Autodesk Fusion 360 part; units mm, degrees
note: some values were not read from the file. Set by a fixed rule: which sketch regions a step uses.
(part 2 of 2)
sketch "bottom inner" plane through (0, 3.175, 0) normal (0, 1, 0) x (-1, 0, 0)
  line L0 (-22.86, -3.175) -> (-24.3417, -3.175)
  line L1 (-24.3417, -3.175) -> (-24.3417, -4.8013)
  arc A0 (-32.8083, -4.8013) -> (-24.3417, -4.8013) centre (-28.575, -4.8013) ccw
  line L2 (-32.8083, -4.8013) -> (-32.8083, -3.175)
  line L3 (-32.8083, -3.175) -> (-53.975, -3.175)
  line L4 (-53.975, -3.175) -> (-53.975, -88.9)
  line L5 (-53.975, -88.9) -> (-32.8083, -88.9)
  line L6 (-32.8083, -88.9) -> (-32.8083, -87.2737)
  arc A1 (-24.3417, -87.2737) -> (-32.8083, -87.2737) centre (-28.575, -87.2737) ccw
  line L7 (-24.3417, -87.2737) -> (-24.3417, -88.9)
  line L8 (-24.3417, -88.9) -> (-3.175, -88.9)
  line L9 (-3.175, -88.9) -> (-3.175, -3.175)
  line L10 (-3.175, -3.175) -> (-7.62, -3.175)
  line L11 (-7.62, -3.175) -> (-7.62, 0)
  line L12 (-7.62, 0) -> (-22.86, 0)
  line L13 (-22.86, 0) -> (-22.86, -3.175)
  spline S0 degree 3 poles (-12.8176, -66.9854) (-12.904, -65.2247) (-13.5003, -63.4767) (-14.5669, -61.8591) knots 0 0 0 0 1 1 1 1
  spline S1 degree 3 poles (-14.5669, -61.8591) (-15.5301, -60.4001) (-16.8758, -59.1069) (-18.9651, -57.638) knots 0 0 0 0 1 1 1 1
  spline S2 degree 3 poles (-18.9651, -57.638) (-20.4751, -56.5756) (-21.3505, -55.9099) (-21.7145, -55.5472) knots 0 0 0 0 1 1 1 1
  spline S3 degree 3 poles (-21.7145, -55.5472) (-22.6537, -54.6081) (-23.284, -53.0854) (-23.7954, -50.5229) knots 0 0 0 0 1 1 1 1
  spline S4 degree 3 poles (-23.7954, -50.5229) (-23.8903, -50.0428) (-23.9837, -49.5059) (-24.1141, -48.6787) knots 0 0 0 0 1 1 1 1
  spline S5 degree 3 poles (-24.1141, -48.6787) (-24.3634, -47.1007) (-24.4795, -46.6673) (-24.6552, -46.6673) knots 0 0 0 0 1 1 1 1
  spline S6 degree 3 poles (-24.6552, -46.6673) (-24.8181, -46.6673) (-24.8521, -46.8953) (-24.8393, -47.8854) knots 0 0 0 0 1 1 1 1
  spline S7 degree 3 poles (-24.8393, -47.8854) (-24.8308, -48.5059) (-24.8209, -48.7254) (-24.7727, -49.4082) knots 0 0 0 0 1 1 1 1
  spline S8 degree 3 poles (-24.7727, -49.4082) (-24.6821, -50.6674) (-24.5574, -51.5626) (-24.3393, -52.5174) knots 0 0 0 0 1 1 1 1
  spline S9 degree 3 poles (-24.3393, -52.5174) (-23.9894, -54.0358) (-23.4724, -55.2314) (-22.8817, -55.8844) knots 0 0 0 0 1 1 1 1
  spline S10 degree 3 poles (-22.8817, -55.8844) (-22.5644, -56.2356) (-21.6097, -56.9666) (-20.4524, -57.7485) knots 0 0 0 0 1 1 1 1
  spline S11 degree 3 poles (-20.4524, -57.7485) (-19.8221, -58.1748) (-19.4708, -58.4227) (-19.0997, -58.7003) knots 0 0 0 0 1 1 1 1
  spline S12 degree 3 poles (-19.0997, -58.7003) (-17.6733, -59.7726) (-16.6548, -60.7967) (-15.8913, -61.9299) knots 0 0 0 0 1 1 1 1
  spline S13 degree 3 poles (-15.8913, -61.9299) (-15.006, -63.2459) (-14.4352, -64.6043) (-14.2128, -65.9244) knots 0 0 0 0 1 1 1 1
  spline S14 degree 3 poles (-14.2128, -65.9244) (-14.0372, -66.9741) (-14.0896, -67.9543) (-14.3714, -68.8282) knots 0 0 0 0 1 1 1 1
  spline S15 degree 3 poles (-14.3714, -68.8282) (-14.591, -69.5082) (-14.9352, -70.079) (-15.4154, -70.5564) knots 0 0 0 0 1 1 1 1
  spline S16 degree 3 poles (-15.4154, -70.5564) (-15.6321, -70.7731) (-15.7752, -70.8892) (-16.0188, -71.0521) knots 0 0 0 0 1 1 1 1
  spline S17 degree 3 poles (-16.0188, -71.0521) (-16.6279, -71.4572) (-17.3007, -71.6924) (-18.1365, -71.7901) knots 0 0 0 0 1 1 1 1
  spline S18 degree 3 poles (-18.1365, -71.7901) (-18.441, -71.827) (-19.162, -71.827) (-19.4396, -71.7915) knots 0 0 0 0 1 1 1 1
  spline S19 degree 3 poles (-19.4396, -71.7915) (-21.0176, -71.5876) (-22.8449, -70.6923) (-24.4087, -69.3552) knots 0 0 0 0 1 1 1 1
  spline S20 degree 3 poles (-24.4087, -69.3552) (-24.6452, -69.154) (-25.1283, -68.6823) (-25.3252, -68.46) knots 0 0 0 0 1 1 1 1
  spline S21 degree 3 poles (-25.3252, -68.46) (-25.8025, -67.9217) (-26.1722, -67.3636) (-26.379, -66.8692) knots 0 0 0 0 1 1 1 1
  line L14 (-26.379, -66.8692) -> (-26.4173, -66.78)
  line L15 (-26.4173, -66.78) -> (-26.304, -66.5505)
  spline S22 degree 3 poles (-26.304, -66.5505) (-26.1793, -66.2984) (-26.1141, -66.1312) (-26.0391, -65.8706) knots 0 0 0 0 1 1 1 1
  spline S23 degree 3 poles (-26.0391, -65.8706) (-25.8096, -65.0717) (-25.7558, -63.964) (-25.9144, -63.2558) knots 0 0 0 0 1 1 1 1
  spline S24 degree 3 poles (-25.9144, -63.2558) (-25.9654, -63.0277) (-26.0334, -62.8422) (-26.1595, -62.5815) knots 0 0 0 0 1 1 1 1
  spline S25 degree 3 poles (-26.1595, -62.5815) (-26.4116, -62.0631) (-26.7771, -61.5319) (-27.0165, -61.3407) knots 0 0 0 0 1 1 1 1
  spline S26 degree 3 poles (-27.0165, -61.3407) (-27.1227, -61.2543) (-27.2332, -61.2217) (-27.389, -61.2316) knots 0 0 0 0 1 1 1 1
  spline S27 degree 3 poles (-27.389, -61.2316) (-27.593, -61.2444) (-27.7502, -61.3648) (-27.8777, -61.6056) knots 0 0 0 0 1 1 1 1
  spline S28 degree 3 poles (-27.8777, -61.6056) (-28.042, -61.9186) (-28.1227, -62.3166) (-28.1397, -62.9002) knots 0 0 0 0 1 1 1 1
  spline S29 degree 3 poles (-28.1397, -62.9002) (-28.1553, -63.447) (-28.0873, -64.0915) (-27.9513, -64.7063) knots 0 0 0 0 1 1 1 1
  spline S30 degree 3 poles (-27.9513, -64.7063) (-27.855, -65.1411) (-27.5915, -66.1808) (-27.5207, -66.4103) knots 0 0 0 0 1 1 1 1
  spline S31 degree 3 poles (-27.5207, -66.4103) (-27.4357, -66.6851) (-27.4244, -66.644) (-27.6397, -66.8593) knots 0 0 0 0 1 1 1 1
  spline S32 degree 3 poles (-27.6397, -66.8593) (-28.0774, -67.2956) (-28.7757, -67.6809) (-29.8763, -68.0903) knots 0 0 0 0 1 1 1 1
  spline S33 degree 3 poles (-29.8763, -68.0903) (-30.4599, -68.307) (-30.6455, -68.3594) (-31.0336, -68.416) knots 0 0 0 0 1 1 1 1
  spline S34 degree 3 poles (-31.0336, -68.416) (-32.0832, -68.569) (-33.8694, -68.5223) (-35.1556, -68.3098) knots 0 0 0 0 1 1 1 1
  spline S35 degree 3 poles (-35.1556, -68.3098) (-35.6202, -68.2333) (-35.8681, -68.171) (-36.2817, -68.0251) knots 0 0 0 0 1 1 1 1
  spline S36 degree 3 poles (-36.2817, -68.0251) (-38.1416, -67.3707) (-39.8314, -66.2177) (-40.5808, -65.0915) knots 0 0 0 0 1 1 1 1
  spline S37 degree 3 poles (-40.5808, -65.0915) (-41.0114, -64.4442) (-41.3839, -63.2175) (-41.5326, -61.9512) knots 0 0 0 0 1 1 1 1
  spline S38 degree 3 poles (-41.5326, -61.9512) (-41.561, -61.7061) (-41.5652, -61.6084) (-41.5652, -61.0871) knots 0 0 0 0 1 1 1 1
  spline S39 degree 3 poles (-41.5652, -61.0871) (-41.5652, -60.4894) (-41.5581, -60.369) (-41.5001, -59.8973) knots 0 0 0 0 1 1 1 1
  spline S40 degree 3 poles (-41.5001, -59.8973) (-41.2522, -57.8944) (-40.3626, -56.3405) (-38.9872, -55.5047) knots 0 0 0 0 1 1 1 1
  spline S41 degree 3 poles (-38.9872, -55.5047) (-38.7846, -55.3815) (-38.279, -55.1336) (-38.0835, -55.0614) knots 0 0 0 0 1 1 1 1
  spline S42 degree 3 poles (-38.0835, -55.0614) (-37.7676, -54.9438) (-37.5509, -54.9041) (-37.0778, -54.8801) knots 0 0 0 0 1 1 1 1
  spline S43 degree 3 poles (-37.0778, -54.8801) (-36.5537, -54.8532) (-36.2166, -54.8857) (-35.293, -55.0515) knots 0 0 0 0 1 1 1 1
  spline S44 degree 3 poles (-35.293, -55.0515) (-34.4573, -55.203) (-34.1343, -55.2342) (-33.8439, -55.1931) knots 0 0 0 0 1 1 1 1
  spline S45 degree 3 poles (-33.8439, -55.1931) (-33.6145, -55.162) (-33.4955, -55.0925) (-33.2561, -54.8546) knots 0 0 0 0 1 1 1 1
  spline S46 degree 3 poles (-33.2561, -54.8546) (-33.0535, -54.6534) (-33.0025, -54.5642) (-33.0025, -54.414) knots 0 0 0 0 1 1 1 1
  spline S47 degree 3 poles (-33.0025, -54.414) (-33.0025, -54.1817) (-33.1952, -53.7851) (-33.5054, -53.3814) knots 0 0 0 0 1 1 1 1
  spline S48 degree 3 poles (-33.5054, -53.3814) (-33.5564, -53.3148) (-33.5975, -53.2568) (-33.5975, -53.2511) knots 0 0 0 0 1 1 1 1
  spline S49 degree 3 poles (-33.5975, -53.2511) (-33.5975, -53.227) (-33.4785, -53.1817) (-33.3609, -53.1619) knots 0 0 0 0 1 1 1 1
  spline S50 degree 3 poles (-33.3609, -53.1619) (-33.2901, -53.1491) (-33.0719, -53.135) (-32.8538, -53.1265) knots 0 0 0 0 1 1 1 1
  spline S51 degree 3 poles (-32.8538, -53.1265) (-32.3552, -53.1095) (-32.1583, -53.074) (-31.9218, -52.9551) knots 0 0 0 0 1 1 1 1
  spline S52 degree 3 poles (-31.9218, -52.9551) (-31.6144, -52.8007) (-31.3622, -52.5018) (-31.2121, -52.1137) knots 0 0 0 0 1 1 1 1
  spline S53 degree 3 poles (-31.2121, -52.1137) (-31.1384, -51.921) (-31.1144, -51.7893) (-31.1144, -51.5683) knots 0 0 0 0 1 1 1 1
  spline S54 degree 3 poles (-31.1144, -51.5683) (-31.1158, -51.3417) (-31.1455, -51.1759) (-31.2319, -50.9238) knots 0 0 0 0 1 1 1 1
  spline S55 degree 3 poles (-31.2319, -50.9238) (-31.3183, -50.6773) (-31.3835, -50.5569) (-31.5407, -50.3657) knots 0 0 0 0 1 1 1 1
  spline S56 degree 3 poles (-31.5407, -50.3657) (-31.5818, -50.3161) (-31.6101, -50.2708) (-31.6045, -50.2651) knots 0 0 0 0 1 1 1 1
  spline S57 degree 3 poles (-31.6045, -50.2651) (-31.5988, -50.2595) (-31.5336, -50.2156) (-31.4614, -50.166) knots 0 0 0 0 1 1 1 1
  spline S58 degree 3 poles (-31.4614, -50.166) (-30.9741, -49.8359) (-31.0166, -49.3473) (-31.5804, -48.8062) knots 0 0 0 0 1 1 1 1
  spline S59 degree 3 poles (-31.5804, -48.8062) (-31.807, -48.588) (-32.0563, -48.401) (-32.4855, -48.1248) knots 0 0 0 0 1 1 1 1
  spline S60 degree 3 poles (-32.4855, -48.1248) (-32.7929, -47.9294) (-32.9147, -47.8344) (-33.0734, -47.673) knots 0 0 0 0 1 1 1 1
  spline S61 degree 3 poles (-33.0734, -47.673) (-33.2164, -47.5285) (-33.283, -47.4307) (-33.3283, -47.3004) knots 0 0 0 0 1 1 1 1
  spline S62 degree 3 poles (-33.3283, -47.3004) (-33.4062, -47.078) (-33.3085, -46.8812) (-33.0578, -46.7622) knots 0 0 0 0 1 1 1 1
  spline S63 degree 3 poles (-33.0578, -46.7622) (-32.8283, -46.6517) (-32.6583, -46.6262) (-32.096, -46.6106) knots 0 0 0 0 1 1 1 1
  spline S64 degree 3 poles (-32.096, -46.6106) (-31.841, -46.6035) (-31.6243, -46.5908) (-31.5903, -46.5823) knots 0 0 0 0 1 1 1 1
  spline S65 degree 3 poles (-31.5903, -46.5823) (-31.4727, -46.5483) (-31.4302, -46.4562) (-31.4302, -46.2366) knots 0 0 0 0 1 1 1 1
  spline S66 degree 3 poles (-31.4302, -46.2366) (-31.4302, -46.0058) (-31.477, -45.8726) (-31.596, -45.7593) knots 0 0 0 0 1 1 1 1
  spline S67 degree 3 poles (-31.596, -45.7593) (-31.688, -45.6715) (-31.7872, -45.6049) (-32.0818, -45.4406) knots 0 0 0 0 1 1 1 1
  spline S68 degree 3 poles (-32.0818, -45.4406) (-32.341, -45.2961) (-32.6371, -45.1091) (-32.783, -44.9986) knots 0 0 0 0 1 1 1 1
  spline S69 degree 3 poles (-32.783, -44.9986) (-32.9218, -44.8924) (-33.1513, -44.6601) (-33.2263, -44.551) knots 0 0 0 0 1 1 1 1
  spline S70 degree 3 poles (-33.2263, -44.551) (-33.3793, -44.3301) (-33.4204, -44.204) (-33.4204, -43.9618) knots 0 0 0 0 1 1 1 1
  spline S71 degree 3 poles (-33.4204, -43.9618) (-33.419, -43.8329) (-33.4119, -43.762) (-33.3935, -43.6997) knots 0 0 0 0 1 1 1 1
  spline S72 degree 3 poles (-33.3935, -43.6997) (-33.2915, -43.3583) (-33.0394, -43.1898) (-32.4784, -43.0835) knots 0 0 0 0 1 1 1 1
  spline S73 degree 3 poles (-32.4784, -43.0835) (-32.147, -43.0212) (-31.9317, -42.9362) (-31.7929, -42.8116) knots 0 0 0 0 1 1 1 1
  spline S74 degree 3 poles (-31.7929, -42.8116) (-31.5832, -42.6246) (-31.5903, -42.364) (-31.8113, -42.16) knots 0 0 0 0 1 1 1 1
  spline S75 degree 3 poles (-31.8113, -42.16) (-31.977, -42.0056) (-32.2532, -41.8243) (-32.7122, -41.5679) knots 0 0 0 0 1 1 1 1
  spline S76 degree 3 poles (-32.7122, -41.5679) (-33.0875, -41.3583) (-33.2717, -41.2393) (-33.3921, -41.1274) knots 0 0 0 0 1 1 1 1
  spline S77 degree 3 poles (-33.3921, -41.1274) (-33.5408, -40.9871) (-33.5451, -40.9135) (-33.4077, -40.8512) knots 0 0 0 0 1 1 1 1
  spline S78 degree 3 poles (-33.4077, -40.8512) (-33.2858, -40.7959) (-33.0946, -40.7747) (-32.5634, -40.7605) knots 0 0 0 0 1 1 1 1
  spline S79 degree 3 poles (-32.5634, -40.7605) (-32.2943, -40.7534) (-32.0209, -40.7407) (-31.9543, -40.7322) knots 0 0 0 0 1 1 1 1
  spline S80 degree 3 poles (-31.9543, -40.7322) (-31.4926, -40.6727) (-31.2815, -40.565) (-31.2631, -40.3795) knots 0 0 0 0 1 1 1 1
  spline S81 degree 3 poles (-31.2631, -40.3795) (-31.2447, -40.1882) (-31.4203, -39.9531) (-31.841, -39.599) knots 0 0 0 0 1 1 1 1
  spline S82 degree 3 poles (-31.841, -39.599) (-32.5082, -39.038) (-33.2462, -38.1329) (-33.5776, -37.4672) knots 0 0 0 0 1 1 1 1
  spline S83 degree 3 poles (-33.5776, -37.4672) (-33.7122, -37.1938) (-33.7448, -37.0748) (-33.7363, -36.8666) knots 0 0 0 0 1 1 1 1
  spline S84 degree 3 poles (-33.7363, -36.8666) (-33.732, -36.7575) (-33.7207, -36.6952) (-33.698, -36.6371) knots 0 0 0 0 1 1 1 1
  spline S85 degree 3 poles (-33.698, -36.6371) (-33.6074, -36.4034) (-33.3496, -36.2787) (-33.1059, -36.3524) knots 0 0 0 0 1 1 1 1
  spline S86 degree 3 poles (-33.1059, -36.3524) (-32.8113, -36.443) (-32.4317, -36.8354) (-32.2051, -37.283) knots 0 0 0 0 1 1 1 1
  spline S87 degree 3 poles (-32.2051, -37.283) (-32.1243, -37.4431) (-32.096, -37.5153) (-32.0096, -37.7788) knots 0 0 0 0 1 1 1 1
  spline S88 degree 3 poles (-32.0096, -37.7788) (-31.8778, -38.1811) (-31.7419, -38.4545) (-31.613, -38.5706) knots 0 0 0 0 1 1 1 1
  spline S89 degree 3 poles (-31.613, -38.5706) (-31.4996, -38.6726) (-31.3792, -38.725) (-31.2404, -38.7321) knots 0 0 0 0 1 1 1 1
  spline S90 degree 3 poles (-31.2404, -38.7321) (-31.0534, -38.742) (-30.9628, -38.6797) (-30.9628, -38.5409) knots 0 0 0 0 1 1 1 1
  spline S91 degree 3 poles (-30.9628, -38.5409) (-30.9628, -38.2406) (-31.6002, -36.6102) (-31.9274, -36.0762) knots 0 0 0 0 1 1 1 1
  spline S92 degree 3 poles (-31.9274, -36.0762) (-32.1399, -35.7277) (-32.4544, -35.4331) (-32.7801, -35.273) knots 0 0 0 0 1 1 1 1
  spline S93 degree 3 poles (-32.7801, -35.273) (-33.3212, -35.0081) (-33.8935, -35.0775) (-34.3015, -35.4543) knots 0 0 0 0 1 1 1 1
  spline S94 degree 3 poles (-34.3015, -35.4543) (-34.6442, -35.773) (-34.7774, -36.1895) (-34.7321, -36.8085) knots 0 0 0 0 1 1 1 1
  spline S95 degree 3 poles (-34.7321, -36.8085) (-34.6967, -37.3) (-34.5947, -37.6612) (-34.368, -38.0975) knots 0 0 0 0 1 1 1 1
  spline S96 degree 3 poles (-34.368, -38.0975) (-34.1825, -38.4545) (-33.9573, -38.7647) (-33.4771, -39.3298) knots 0 0 0 0 1 1 1 1
  spline S97 degree 3 poles (-33.4771, -39.3298) (-33.1173, -39.7534) (-33.0535, -39.8341) (-33.0649, -39.8511) knots 0 0 0 0 1 1 1 1
  spline S98 degree 3 poles (-33.0649, -39.8511) (-33.0691, -39.8582) (-33.1286, -39.8695) (-33.1966, -39.8738) knots 0 0 0 0 1 1 1 1
  spline S99 degree 3 poles (-33.1966, -39.8738) (-33.6895, -39.9134) (-33.9898, -40.0197) (-34.208, -40.2364) knots 0 0 0 0 1 1 1 1
  spline S100 degree 3 poles (-34.208, -40.2364) (-34.3794, -40.405) (-34.453, -40.5792) (-34.4516, -40.8172) knots 0 0 0 0 1 1 1 1
  spline S101 degree 3 poles (-34.4516, -40.8172) (-34.4516, -41.0381) (-34.3794, -41.2492) (-34.2292, -41.4744) knots 0 0 0 0 1 1 1 1
  spline S102 degree 3 poles (-34.2292, -41.4744) (-34.123, -41.6316) (-34.0068, -41.7563) (-33.7235, -42.0084) knots 0 0 0 0 1 1 1 1
  line L16 (-33.7235, -42.0084) -> (-33.4813, -42.2251)
  line L17 (-33.4813, -42.2251) -> (-33.7136, -42.4518)
  spline S103 degree 3 poles (-33.7136, -42.4518) (-33.9573, -42.6912) (-34.0578, -42.8172) (-34.1527, -43.0056) knots 0 0 0 0 1 1 1 1
  spline S104 degree 3 poles (-34.1527, -43.0056) (-34.293, -43.2804) (-34.3411, -43.5212) (-34.3298, -43.8683) knots 0 0 0 0 1 1 1 1
  spline S105 degree 3 poles (-34.3298, -43.8683) (-34.3185, -44.1785) (-34.266, -44.3995) (-34.1286, -44.6913) knots 0 0 0 0 1 1 1 1
  spline S106 degree 3 poles (-34.1286, -44.6913) (-34.0111, -44.9434) (-33.8793, -45.1332) (-33.5861, -45.4703) knots 0 0 0 0 1 1 1 1
  spline S107 degree 3 poles (-33.5861, -45.4703) (-33.3949, -45.6899) (-33.3637, -45.7352) (-33.3836, -45.772) knots 0 0 0 0 1 1 1 1
  spline S108 degree 3 poles (-33.3836, -45.772) (-33.3907, -45.7862) (-33.4941, -45.8868) (-33.6116, -45.993) knots 0 0 0 0 1 1 1 1
  spline S109 degree 3 poles (-33.6116, -45.993) (-33.9997, -46.3471) (-34.174, -46.5922) (-34.266, -46.9166) knots 0 0 0 0 1 1 1 1
  spline S110 degree 3 poles (-34.266, -46.9166) (-34.3057, -47.061) (-34.3085, -47.3203) (-34.2717, -47.4605) knots 0 0 0 0 1 1 1 1
  spline S111 degree 3 poles (-34.2717, -47.4605) (-34.2363, -47.5951) (-34.1343, -47.7962) (-34.0366, -47.9251) knots 0 0 0 0 1 1 1 1
  spline S112 degree 3 poles (-34.0366, -47.9251) (-33.8793, -48.1333) (-33.5946, -48.3741) (-33.2957, -48.5498) knots 0 0 0 0 1 1 1 1
  spline S113 degree 3 poles (-33.2957, -48.5498) (-33.2278, -48.5894) (-33.1173, -48.6546) (-33.0479, -48.6943) knots 0 0 0 0 1 1 1 1
  spline S114 degree 3 poles (-33.0479, -48.6943) (-32.7306, -48.8812) (-32.4048, -49.1631) (-32.3184, -49.3274) knots 0 0 0 0 1 1 1 1
  line L18 (-32.3184, -49.3274) -> (-32.2787, -49.4011)
  line L19 (-32.2787, -49.4011) -> (-32.3325, -49.4266)
  spline S115 degree 3 poles (-32.3325, -49.4266) (-32.3821, -49.4492) (-32.4629, -49.4507) (-33.2858, -49.4507) knots 0 0 0 0 1 1 1 1
  spline S116 degree 3 poles (-33.2858, -49.4507) (-34.1598, -49.4507) (-34.1867, -49.4521) (-34.2335, -49.479) knots 0 0 0 0 1 1 1 1
  spline S117 degree 3 poles (-34.2335, -49.479) (-34.327, -49.5342) (-34.361, -49.615) (-34.3624, -49.7835) knots 0 0 0 0 1 1 1 1
  spline S118 degree 3 poles (-34.3624, -49.7835) (-34.3638, -50.0555) (-34.2051, -50.1532) (-33.5451, -50.2864) knots 0 0 0 0 1 1 1 1
  spline S119 degree 3 poles (-33.5451, -50.2864) (-33.0974, -50.377) (-32.9218, -50.4309) (-32.6852, -50.5527) knots 0 0 0 0 1 1 1 1
  spline S120 degree 3 poles (-32.6852, -50.5527) (-32.3538, -50.7227) (-32.1427, -50.9493) (-32.0747, -51.2099) knots 0 0 0 0 1 1 1 1
  spline S121 degree 3 poles (-32.0747, -51.2099) (-32.0025, -51.4847) (-32.1243, -51.7709) (-32.3835, -51.9338) knots 0 0 0 0 1 1 1 1
  spline S122 degree 3 poles (-32.3835, -51.9338) (-32.5408, -52.0329) (-32.7107, -52.0882) (-32.9742, -52.1278) knots 0 0 0 0 1 1 1 1
  spline S123 degree 3 poles (-32.9742, -52.1278) (-33.606, -52.2227) (-33.9459, -52.3516) (-34.1655, -52.5825) knots 0 0 0 0 1 1 1 1
  spline S124 degree 3 poles (-34.1655, -52.5825) (-34.31, -52.7355) (-34.4034, -52.948) (-34.4148, -53.1562) knots 0 0 0 0 1 1 1 1
  spline S125 degree 3 poles (-34.4148, -53.1562) (-34.4247, -53.3078) (-34.4049, -53.3814) (-34.2845, -53.6364) knots 0 0 0 0 1 1 1 1
  spline S126 degree 3 poles (-34.2845, -53.6364) (-34.2363, -53.7412) (-34.1811, -53.8715) (-34.1655, -53.9268) knots 0 0 0 0 1 1 1 1
  spline S127 degree 3 poles (-34.1655, -53.9268) (-34.1371, -54.0188) (-34.1216, -54.1647) (-34.1386, -54.1817) knots 0 0 0 0 1 1 1 1
  spline S128 degree 3 poles (-34.1386, -54.1817) (-34.1513, -54.1945) (-34.5635, -54.084) (-34.7958, -54.0075) knots 0 0 0 0 1 1 1 1
  spline S129 degree 3 poles (-34.7958, -54.0075) (-35.0621, -53.9183) (-35.2803, -53.8616) (-35.5805, -53.8078) knots 0 0 0 0 1 1 1 1
  spline S130 degree 3 poles (-35.5805, -53.8078) (-36.361, -53.6647) (-36.8951, -53.6435) (-37.5353, -53.7299) knots 0 0 0 0 1 1 1 1
  spline S131 degree 3 poles (-37.5353, -53.7299) (-37.9192, -53.7809) (-38.3767, -53.8956) (-38.7535, -54.0344) knots 0 0 0 0 1 1 1 1
  spline S132 degree 3 poles (-38.7535, -54.0344) (-39.0269, -54.135) (-39.449, -54.3489) (-39.6742, -54.4976) knots 0 0 0 0 1 1 1 1
  spline S133 degree 3 poles (-39.6742, -54.4976) (-40.1218, -54.7951) (-40.5978, -55.2625) (-40.9958, -55.7965) knots 0 0 0 0 1 1 1 1
  spline S134 degree 3 poles (-40.9958, -55.7965) (-41.5992, -56.6054) (-42.0709, -57.5785) (-42.357, -58.6111) knots 0 0 0 0 1 1 1 1
  spline S135 degree 3 poles (-42.357, -58.6111) (-42.561, -59.3434) (-42.6531, -60.1707) (-42.6531, -61.2642) knots 0 0 0 0 1 1 1 1
  spline S136 degree 3 poles (-42.6531, -61.2642) (-42.6531, -62.1849) (-42.5879, -62.8209) (-42.4364, -63.3719) knots 0 0 0 0 1 1 1 1
  spline S137 degree 3 poles (-42.4364, -63.3719) (-42.2026, -64.2232) (-41.7437, -65.1624) (-41.1672, -65.9669) knots 0 0 0 0 1 1 1 1
  spline S138 degree 3 poles (-41.1672, -65.9669) (-40.5014, -66.899) (-39.7139, -67.6526) (-38.8852, -68.1497) knots 0 0 0 0 1 1 1 1
  spline S139 degree 3 poles (-38.8852, -68.1497) (-37.3101, -69.0945) (-34.0791, -69.8821) (-32.1668, -69.7858) knots 0 0 0 0 1 1 1 1
  spline S140 degree 3 poles (-32.1668, -69.7858) (-30.984, -69.7263) (-29.9047, -69.4444) (-28.8664, -68.9246) knots 0 0 0 0 1 1 1 1
  spline S141 degree 3 poles (-28.8664, -68.9246) (-28.3919, -68.688) (-28.0448, -68.4685) (-27.6624, -68.1625) knots 0 0 0 0 1 1 1 1
  spline S142 degree 3 poles (-27.6624, -68.1625) (-27.5646, -68.0846) (-27.4244, -67.9741) (-27.3507, -67.916) knots 0 0 0 0 1 1 1 1
  spline S143 degree 3 poles (-27.3507, -67.916) (-27.2771, -67.8579) (-27.1708, -67.7701) (-27.1156, -67.7205) knots 0 0 0 0 1 1 1 1
  spline S144 degree 3 poles (-27.1156, -67.7205) (-27.0589, -67.6724) (-27.0108, -67.6313) (-27.0065, -67.6313) knots 0 0 0 0 1 1 1 1
  spline S145 degree 3 poles (-27.0065, -67.6313) (-26.9995, -67.6313) (-26.3776, -68.4444) (-25.998, -68.9472) knots 0 0 0 0 1 1 1 1
  spline S146 degree 3 poles (-25.998, -68.9472) (-25.5022, -69.6087) (-24.8039, -70.2334) (-23.8676, -70.8595) knots 0 0 0 0 1 1 1 1
  spline S147 degree 3 poles (-23.8676, -70.8595) (-22.3066, -71.9006) (-20.5544, -72.6259) (-19.1776, -72.8001) knots 0 0 0 0 1 1 1 1
  spline S148 degree 3 poles (-19.1776, -72.8001) (-17.2526, -73.0451) (-15.2553, -72.4403) (-14.1476, -71.2759) knots 0 0 0 0 1 1 1 1
  spline S149 degree 3 poles (-14.1476, -71.2759) (-13.3983, -70.487) (-12.9394, -69.341) (-12.8331, -67.9854) knots 0 0 0 0 1 1 1 1
  spline S150 degree 3 poles (-12.8331, -67.9854) (-12.8119, -67.7234) (-12.8048, -67.2446) (-12.8176, -66.9854) knots 0 0 0 0 1 1 1 1
  spline S151 degree 3 poles (-26.7147, -64.5731) (-26.7332, -64.8012) (-26.7643, -64.9867) (-26.8266, -65.2219) knots 0 0 0 0 1 1 1 1
  spline S152 degree 3 poles (-26.8266, -65.2219) (-26.8833, -65.4315) (-26.8819, -65.4329) (-26.974, -65.1539) knots 0 0 0 0 1 1 1 1
  spline S153 degree 3 poles (-26.974, -65.1539) (-27.1652, -64.5759) (-27.2714, -63.838) (-27.2728, -63.0773) knots 0 0 0 0 1 1 1 1
  spline S154 degree 3 poles (-27.2728, -63.0773) (-27.2728, -62.7827) (-27.27, -62.7303) (-27.2473, -62.6821) knots 0 0 0 0 1 1 1 1
  spline S155 degree 3 poles (-27.2473, -62.6821) (-27.2247, -62.6311) (-27.2218, -62.6283) (-27.1978, -62.6495) knots 0 0 0 0 1 1 1 1
  spline S156 degree 3 poles (-27.1978, -62.6495) (-27.1298, -62.7104) (-26.94, -63.1439) (-26.8507, -63.4385) knots 0 0 0 0 1 1 1 1
  spline S157 degree 3 poles (-26.8507, -63.4385) (-26.7133, -63.8918) (-26.6807, -64.1595) (-26.7147, -64.5731) knots 0 0 0 0 1 1 1 1
  spline S158 degree 3 poles (-22.0913, -29.7048) (-22.1607, -28.8167) (-22.3279, -28.1282) (-22.6976, -27.1962) knots 0 0 0 0 1 1 1 1
  spline S159 degree 3 poles (-22.6976, -27.1962) (-23.6353, -24.8392) (-25.3407, -22.645) (-27.4641, -21.0685) knots 0 0 0 0 1 1 1 1
  spline S160 degree 3 poles (-27.4641, -21.0685) (-27.9641, -20.6973) (-28.212, -20.5444) (-28.8026, -20.2412) knots 0 0 0 0 1 1 1 1
  spline S161 degree 3 poles (-28.8026, -20.2412) (-30.6625, -19.2865) (-32.2603, -18.9763) (-33.6187, -19.3035) knots 0 0 0 0 1 1 1 1
  spline S162 degree 3 poles (-33.6187, -19.3035) (-35.3043, -19.7086) (-36.548, -21.0557) (-37.2704, -23.2598) knots 0 0 0 0 1 1 1 1
  spline S163 degree 3 poles (-37.2704, -23.2598) (-37.5466, -24.1026) (-37.6274, -24.6295) (-37.6444, -25.7174) knots 0 0 0 0 1 1 1 1
  spline S164 degree 3 poles (-37.6444, -25.7174) (-37.6557, -26.4185) (-37.6245, -27.0064) (-37.5495, -27.5843) knots 0 0 0 0 1 1 1 1
  spline S165 degree 3 poles (-37.5495, -27.5843) (-37.473, -28.1622) (-37.3781, -28.5305) (-37.1444, -29.1694) knots 0 0 0 0 1 1 1 1
  spline S166 degree 3 poles (-37.1444, -29.1694) (-36.6429, -30.5349) (-35.9757, -31.5448) (-34.9176, -32.5406) knots 0 0 0 0 1 1 1 1
  spline S167 degree 3 poles (-34.9176, -32.5406) (-34.1966, -33.2177) (-33.6541, -33.5831) (-33.1626, -33.7205) knots 0 0 0 0 1 1 1 1
  spline S168 degree 3 poles (-33.1626, -33.7205) (-32.766, -33.8324) (-32.4317, -33.8806) (-32.0393, -33.8806) knots 0 0 0 0 1 1 1 1
  spline S169 degree 3 poles (-32.0393, -33.8806) (-31.6441, -33.882) (-31.3637, -33.8409) (-31.0407, -33.7333) knots 0 0 0 0 1 1 1 1
  spline S170 degree 3 poles (-31.0407, -33.7333) (-30.4968, -33.552) (-30.0577, -33.2205) (-29.7489, -32.7573) knots 0 0 0 0 1 1 1 1
  spline S171 degree 3 poles (-29.7489, -32.7573) (-29.5364, -32.44) (-29.3834, -32.0094) (-29.3267, -31.5774) knots 0 0 0 0 1 1 1 1
  spline S172 degree 3 poles (-29.3267, -31.5774) (-29.2984, -31.3564) (-29.2984, -30.9301) (-29.3282, -30.7332) knots 0 0 0 0 1 1 1 1
  spline S173 degree 3 poles (-29.3282, -30.7332) (-29.4486, -29.9088) (-29.9203, -29.032) (-30.3509, -28.8294) knots 0 0 0 0 1 1 1 1
  spline S174 degree 3 poles (-30.3509, -28.8294) (-30.4288, -28.7926) (-30.4514, -28.7883) (-30.5407, -28.794) knots 0 0 0 0 1 1 1 1
  spline S175 degree 3 poles (-30.5407, -28.794) (-30.671, -28.8011) (-30.6993, -28.8294) (-30.6908, -28.947) knots 0 0 0 0 1 1 1 1
  spline S176 degree 3 poles (-30.6908, -28.947) (-30.6837, -29.0546) (-30.6257, -29.1694) (-30.4514, -29.43) knots 0 0 0 0 1 1 1 1
  spline S177 degree 3 poles (-30.4514, -29.43) (-30.2885, -29.6694) (-30.2092, -29.8394) (-30.1483, -30.0731) knots 0 0 0 0 1 1 1 1
  spline S178 degree 3 poles (-30.1483, -30.0731) (-29.9712, -30.7572) (-30.1001, -31.6241) (-30.4684, -32.2304) knots 0 0 0 0 1 1 1 1
  spline S179 degree 3 poles (-30.4684, -32.2304) (-30.7673, -32.7177) (-31.1129, -32.9216) (-31.6923, -32.9514) knots 0 0 0 0 1 1 1 1
  spline S180 degree 3 poles (-31.6923, -32.9514) (-31.7858, -32.9556) (-31.9416, -32.9514) (-32.0393, -32.9429) knots 0 0 0 0 1 1 1 1
  spline S181 degree 3 poles (-32.0393, -32.9429) (-32.834, -32.8692) (-33.4983, -32.5279) (-34.2901, -31.7828) knots 0 0 0 0 1 1 1 1
  spline S182 degree 3 poles (-34.2901, -31.7828) (-35.4177, -30.7233) (-36.1882, -29.2133) (-36.4715, -27.5092) knots 0 0 0 0 1 1 1 1
  spline S183 degree 3 poles (-36.4715, -27.5092) (-36.565, -26.9469) (-36.5919, -26.563) (-36.582, -25.9242) knots 0 0 0 0 1 1 1 1
  spline S184 degree 3 poles (-36.582, -25.9242) (-36.5721, -25.325) (-36.5353, -24.9511) (-36.429, -24.4213) knots 0 0 0 0 1 1 1 1
  spline S185 degree 3 poles (-36.429, -24.4213) (-36.2279, -23.4085) (-35.8327, -22.4566) (-35.2831, -21.662) knots 0 0 0 0 1 1 1 1
  spline S186 degree 3 poles (-35.2831, -21.662) (-34.8766, -21.0727) (-34.0805, -20.5344) (-33.1994, -20.2526) knots 0 0 0 0 1 1 1 1
  spline S187 degree 3 poles (-33.1994, -20.2526) (-32.8425, -20.1392) (-32.5634, -20.0939) (-32.1951, -20.0939) knots 0 0 0 0 1 1 1 1
  spline S188 degree 3 poles (-32.1951, -20.0939) (-31.9118, -20.0939) (-31.6696, -20.1194) (-31.3722, -20.1789) knots 0 0 0 0 1 1 1 1
  spline S189 degree 3 poles (-31.3722, -20.1789) (-28.933, -20.6704) (-25.8549, -23.281) (-24.1325, -26.3194) knots 0 0 0 0 1 1 1 1
  spline S190 degree 3 poles (-24.1325, -26.3194) (-23.2344, -27.9016) (-22.8151, -29.4796) (-22.9681, -30.6893) knots 0 0 0 0 1 1 1 1
  spline S191 degree 3 poles (-22.9681, -30.6893) (-23.0942, -31.6709) (-23.5786, -32.2786) (-24.3662, -32.4386) knots 0 0 0 0 1 1 1 1
  spline S192 degree 3 poles (-24.3662, -32.4386) (-24.5263, -32.4712) (-24.7954, -32.4811) (-24.9781, -32.4613) knots 0 0 0 0 1 1 1 1
  spline S193 degree 3 poles (-24.9781, -32.4613) (-25.5985, -32.3933) (-26.083, -32.1497) (-26.7558, -31.5618) knots 0 0 0 0 1 1 1 1
  spline S194 degree 3 poles (-26.7558, -31.5618) (-27.1397, -31.2261) (-27.2686, -31.1425) (-27.4003, -31.1425) knots 0 0 0 0 1 1 1 1
  spline S195 degree 3 poles (-27.4003, -31.1425) (-27.4655, -31.1425) (-27.4811, -31.1482) (-27.5051, -31.1794) knots 0 0 0 0 1 1 1 1
  spline S196 degree 3 poles (-27.5051, -31.1794) (-27.5986, -31.2983) (-27.4896, -31.4995) (-27.1567, -31.8239) knots 0 0 0 0 1 1 1 1
  spline S197 degree 3 poles (-27.1567, -31.8239) (-26.4796, -32.4825) (-25.3422, -33.1596) (-24.6821, -33.297) knots 0 0 0 0 1 1 1 1
  spline S198 degree 3 poles (-24.6821, -33.297) (-24.4993, -33.3353) (-24.1891, -33.3395) (-23.9979, -33.3055) knots 0 0 0 0 1 1 1 1
  spline S199 degree 3 poles (-23.9979, -33.3055) (-23.3846, -33.195) (-22.8534, -32.8083) (-22.5729, -32.263) knots 0 0 0 0 1 1 1 1
  spline S200 degree 3 poles (-22.5729, -32.263) (-22.3137, -31.7615) (-22.1437, -31.1255) (-22.0956, -30.4768) knots 0 0 0 0 1 1 1 1
  spline S201 degree 3 poles (-22.0956, -30.4768) (-22.0828, -30.3026) (-22.08, -29.8436) (-22.0913, -29.7048) knots 0 0 0 0 1 1 1 1
extrude "Extrude5" add sketch "bottom inner" along normal blind 0.762 contours S0 S1 S2 S3 S4 S5 S6 S7 S8 S9 S10 S11 S12 S13 S14 S15 S16 S17 S18 S19 S20 S21 L14 L15 S22 S23 S24 S25 S26 S27 S28 S29 S30 S31 S32 S33 S34 S35 S36 S37 S38 S39 S40 S41 S42 S43 S44 S45 S46 S47 S48 S49 S50 S51 S52 S53 S54 S55 S56 S57 S58 S59 S60 S61 S62 S63 S64 S65 S66 S67 S68 S69 S70 S71 S72 S73 S74 S75 S76 S77 S78 S79 S80 S81 S82 S83 S84 S85 S86 S87 S88 S89 S90 S91 S92 S93 S94 S95 S96 S97 S98 S99 S100 S101 S102 L16 L17 S103 S104 S105 S106 S107 S108 S109 S110 S111 S112 S113 S114 L18 L19 S115 S116 S117 S118 S119 S120 S121 S122 S123 S124 S125 S126 S127 S128 S129 S130 S131 S132 S133 S134 S135 S136 S137 S138 S139 S140 S141 S142 S143 S144 S145 S146 S147 S148 S149 S150 | S158 S159 S160 S161 S162 S163 S164 S165 S166 S167 S168 S169 S170 S171 S172 S173 S174 S175 S176 S177 S178 S179 S180 S181 S182 S183 S184 S185 S186 S187 S188 S189 S190 S191 S192 S193 S194 S195 S196 S197 S198 S199 S200 S201
extrude "Extrude6" cut sketch "top2" against normal blind 25.4 contours A8 | A9
extrude "Extrude7" cut sketch "top" against normal up to surface (47.625 mm away) contours L5 L23 L24 L25 A12 A13 L26 L27 A14 A15 L28 L29
extrude "Extrude8" cut sketch "top2" against normal up to surface (25.4 mm away) contours A10 | A13
equation "d1 = 4 1/8\""
equation "d2 = 3 5/8\""
equation "d5 = ( 1 / 8 ) * 1 in"
equation "d6 = ( 1 / 8 ) * 1 in"
equation "d7 = ( 1 / 8 ) * 1 in"
equation "d8 = ( 1 / 8 ) * 1 in"
equation "d9 = ( 1 / 8 ) * 1 in"
equation "d10 = ( 1 / 6 ) * 1 in"
equation "d11 = ( 1 / 6 ) * 1 in"
equation "d12 = ( 1 / 8 ) * 1 in"
equation "d13 = ( 1 / 8 ) * 1 in"
equation "d14 = ( 1 / 8 ) * 1 in"
equation "d15 = ( 1 / 8 ) * 1 in"
equation "d16 = -2 in + ( ( 1 / 8 ) * 1 in )"
equation "d29 = ( 1 / 8 ) * 1 in"
equation "predrill_hole = 0.1 in"
equation "d33 = predrill_hole"
equation "d34 = predrill_hole"
equation "enscription_height = 0.03 in"
equation "d36 = enscription_height"
equation "d38 = enscription_height"
equation "mount_hole_depth = 1 in"
equation "d41 = -mount_hole_depth"
equation "d43 = 3.875 in / 2"
